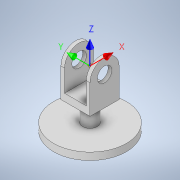
# Autodesk Inventor part: FP
Saved by Autodesk Inventor 2020.1 (Build 241239000, 239)
## iProperties
Created: 2019-10-24
Part Number: FP
Material: Generic
Document SubType Name: Modeling
Designer: sshel
Density: 1 g/cm^3
Appearance: Default
Author: sshel
Autodesk Inventor part; units mm, degrees
ref_plane "YZ Plane" through (0, 0, 0) normal (1, 0, 0) x (0, 1, 0)
ref_plane "XZ Plane" through (0, 0, 0) normal (0, 1, 0) x (-1, 0, 0)
ref_plane "XY Plane" through (0, 0, 0) normal (0, 0, 1) x (1, 0, 0)
sketch "Sketch2" plane through (0, 0, 0) normal (0, 1, 0) x (-1, 0, 0)
  line L0 (0, 143.7774) -> (0, -346.4102) construction
  line L1 (190.8875, 0) -> (-168.3726, 0)
  arc A0 (200, -346.4102) -> (0, 400) centre (0, 0) ccw construction
  line L2 (0, 0) -> (0, -346.4102) construction
  line L3 (0, -1546.4102) -> (1000, -1546.4102)
  line L4 (1000, -1546.4102) -> (1000, -1346.4102)
  line L5 (1000, -1346.4102) -> (200, -1346.4102)
  line L6 (200, -1346.4102) -> (200, -346.4102)
  line L7 (0, 0) -> (0, 400) construction
  line L8 (200, -346.4102) -> (0, -346.4102)
  line L9 (0, -346.4102) -> (0, -95.5661) construction
  line L10 (0, -346.4102) -> (0, -1546.4102)
  dimension "d0" = 400
  dimension "ht" = 1000
  dimension "base_thick" = 200
  dimension "base_radius" = 1000
  dimension "d11" = 200
  constraints: 22 end point, 9 perpendicular, 5 vertical, 2 point on circle, 1 centre point, 1 coincident, 1 point on line
  measures "d0" radius of A0
  measures "ht" distance of L5.end L6.end
  measures "base_thick" distance of L3.end L4.end
  measures "base_radius" distance of L3.start L3.end
  measures "d11" distance between parallel lines of L2 L6
revolve "Revolution2" add sketch "Sketch2" angle 360 about axis through (0, 0, 143.7774) along (0, 0, -1)
sketch "Sketch3" plane through (0, 0, 0) normal (0, 1, 0) x (-1, 0, 0)
  line L0 (68.3369, 0) -> (-71.9882, 0)
  line L1 (0, 52.8788) -> (0, -69.4874)
  arc A0 (400, 0) -> (-400, 0) centre (0, 0) ccw
  line L2 (400, 0) -> (400, -800)
  line L3 (400, -800) -> (-400, -800)
  line L4 (-400, -800) -> (-400, 0)
  dimension "d26" = 400
  dimension "d27" = 800
  constraints: 10 end point, 4 perpendicular, 3 point on line, 2 point on circle, 2 tangent, 1 centre point, 1 coincident, 1 horizontal
  measures "d26" radius of A0
  measures "d27" distance of L3.end L4.end
extrude "Extrusion1" add sketch "Sketch3" along normal mid plane 800
sketch "Sketch4" plane through (0, 0, 0) normal (0, 1, 0) x (-1, 0, 0)
  circle A0 centre (0, 0) radius 200
  dimension "d30" = 200
  constraints: 1 centre point, 1 coincident
  measures "d30" radius of A0
extrude "Extrusion2" cut sketch "Sketch4" along normal through all both and the other way through all
sketch "Sketch5" plane through (0, 0, 0) normal (1, 0, 0) x (0, 1, 0)
  line L0 (300, -600) -> (-300, -600)
  line L1 (-300, -600) -> (-300, 400)
  line L2 (-300, 400) -> (300, 400)
  line L3 (300, 400) -> (300, -600)
  line L4 (0, -62.7821) -> (0, 60)
  line L5 (91.6333, 0) -> (-95.5004, 0)
  line L6 (0, -200) -> (0, 150) construction
  point P0 (0, 0)
  dimension "d35" = 300
  dimension "d36" = 400
  dimension "d39" = 600
  constraints: 12 end point, 2 horizontal, 2 parallel, 2 point on line, 1 perpendicular, 1 vertical, 1 other
  measures "d35" distance between parallel lines of L6 L1
  measures "d36" distance between parallel lines of L5 L2
  measures "d39" distance between parallel lines of L5 L0
extrude "Extrusion3" cut sketch "Sketch5" along normal through all both and the other way through all
equation "\"d0\" = S_radius"
equation "\"ht\" = 5 * rod_radius"
equation "\"base_thick\" = rod_radius"
equation "\"base_radius\" = 5 * rod_radius"
equation "\"d11\" = rod_radius"
equation "\"d26\" = S_radius"
equation "\"d27\" = 2 * S_radius"
equation "\"d28\" = 2 * S_radius"
equation "\"d30\" = rod_radius"
equation "\"d35\" = 1.5 * rod_radius"
equation "\"d36\" = S_radius"
equation "\"d39\" = 1.5 * S_radius"
equation "\"rod_radius\" = 200"
equation "\"S_radius\" = 2 * rod_radius"
body "Solid2"
